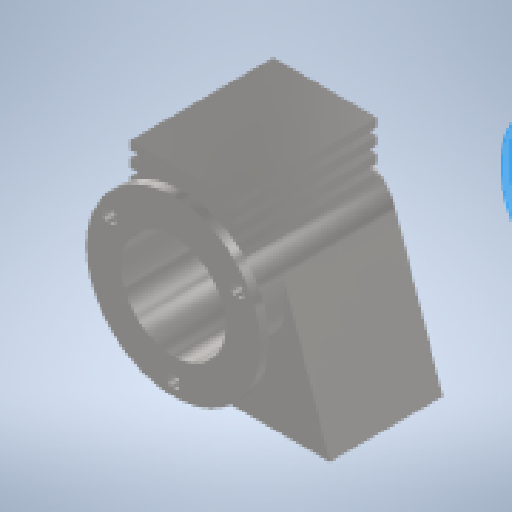
# Autodesk Inventor part: Base do Motor Industrial
Saved by Autodesk Inventor 2023.2 (Build 272271000, 271)
## iProperties
Created: 2022-07-18
Part Number: Base do Motor Industrial
Material: Steel, Carbon
Document SubType Name: Modeling
Designer: coqui
Density: 7.85 g/cm^3
Appearance: Semi-Polished
Mass: 4415.21 g
Surface Area: 866.573 cm^2
Volume: 562.447 cm^3
Author: coqui
Autodesk Inventor part; units mm, degrees
ref_plane "YZ Plane" through (0, 0, 0) normal (1, 0, 0) x (0, 1, 0)
ref_plane "XZ Plane" through (0, 0, 0) normal (0, 1, 0) x (-1, 0, 0)
ref_plane "XY Plane" through (0, 0, 0) normal (0, 0, 1) x (1, 0, 0)
sketch "Sketch1" plane through (0, 0, 0) normal (0, 0, 1) x (1, 0, 0)
  arc A0 (33.1265, 11.2976) -> (-33.1265, 11.2976) centre (0, 0) ccw
  line L0 (-60, -67.5) -> (60, -67.5)
  line L1 (-60, -67.5) -> (-33.1265, 11.2976)
  line L2 (60, -67.5) -> (33.1265, 11.2976)
  point P0 (0, -67.5)
  dimension "d0" = 70
  dimension "d1" = 120
  dimension "d2" = 60
  dimension "d3" = 67.5
  constraints: 6 end point, 2 point on circle, 2 tangent, 1 centre point, 1 coincident, 1 horizontal, 1 midpoint
  measures "d0" diameter of A0
  measures "d1" distance of L0.start L0.end
  measures "d2" horizontal distance of L0.end point (0, 0)
  measures "d3" distance of point (0, -67.5) point (0, 0)
extrude "Extrusion1" add sketch "Sketch1" along normal blind 65
sketch "Sketch2" plane through (0, 0, 65) normal (0, 0, 1) x (1, 0, 0)
  circle A0 centre (0, 0) radius 35
  dimension "d6" = 70
  constraints: 1 centre point, 1 coincident
  measures "d6" diameter of A0
extrude "Extrusion2" add sketch "Sketch2" along normal blind 25
sketch "Sketch3" plane through (0, 0, 90) normal (0, 0, 1) x (1, 0, 0)
  circle A0 centre (0, 0) radius 50
  dimension "d9" = 100
  constraints: 1 centre point, 1 coincident
  measures "d9" diameter of A0
extrude "Extrusion3" add sketch "Sketch3" along normal blind 5
sketch "Sketch4" plane through (0, 0, 95) normal (0, 0, 1) x (1, 0, 0)
  circle A0 centre (0, -42.5) radius 3.75
  circle A1 centre (36.8061, 21.25) radius 3.75
  circle A2 centre (-36.8061, 21.25) radius 3.75
  point P0 (0, 0)
  dimension "d12" = 7.5
  dimension "d13" = 42.5
  dimension "d16" = 360
  constraints: 3 centre point, 7 other
  measures "d12" diameter of A0
  measures "d13" distance of point (0, 0) A0.centre
extrude "Extrusion4" cut sketch "Sketch4" against normal blind 5
sketch "Sketch5" plane through (0, 0, 90) normal (0, 0, -1) x (-1, 0, 0)
  line L0 (0, 60) -> (-30, 60)
  line L1 (-30, 60) -> (-30, 55.5)
  line L2 (-30, 55.5) -> (-25, 55.5)
  line L3 (-25, 55.5) -> (-25, 51)
  line L4 (-25, 51) -> (-30, 51)
  line L5 (-30, 51) -> (-30, 46.5)
  line L6 (-30, 46.5) -> (-25, 46.5)
  line L7 (-25, 46.5) -> (-25, 42)
  line L8 (-25, 42) -> (-30, 42)
  line L9 (-30, 42) -> (-30, 37.5)
  line L10 (-30, 37.5) -> (-25, 37.5)
  line L11 (-25, 37.5) -> (-25, 33)
  line L12 (-25, 33) -> (-30, 33)
  line L13 (-30, 33) -> (-30, 28.5)
  line L14 (-30, 28.5) -> (-25, 28.5)
  line L15 (-25, 28.5) -> (-25, 24)
  line L16 (-25, 24) -> (-30, 24)
  line L17 (-30, 24) -> (-30, 19.5)
  line L18 (-30, 19.5) -> (-25, 19.5)
  arc A0 (33.1265, 11.2976) -> (-33.1265, 11.2976) centre (0, 0) ccw projected
  line L19 (-25, 19.5) -> (0, 19.5)
  line L20 (0, 60) -> (30, 60)
  line L21 (30, 60) -> (30, 55.5)
  line L22 (30, 55.5) -> (25, 55.5)
  line L23 (25, 55.5) -> (25, 51)
  line L24 (25, 51) -> (30, 51)
  line L25 (30, 51) -> (30, 46.5)
  line L26 (30, 46.5) -> (25, 46.5)
  line L27 (25, 46.5) -> (25, 42)
  line L28 (25, 42) -> (30, 42)
  line L29 (30, 42) -> (30, 37.5)
  line L30 (30, 37.5) -> (25, 37.5)
  line L31 (25, 37.5) -> (25, 33)
  line L32 (25, 33) -> (30, 33)
  line L33 (30, 33) -> (30, 28.5)
  line L34 (30, 28.5) -> (25, 28.5)
  line L35 (25, 28.5) -> (25, 24)
  line L36 (25, 24) -> (30, 24)
  line L37 (30, 24) -> (30, 19.5)
  line L38 (30, 19.5) -> (25, 19.5)
  line L39 (25, 19.5) -> (0, 19.5)
  point P0 (0, 35)
  point P1 (-25, 24.4949)
  point P2 (25, 24.4949)
  dimension "d20" = 4.5
  dimension "d21" = 4.5
  dimension "d22" = 4.5
  dimension "d23" = 4.5
  dimension "d24" = 4.5
  dimension "d25" = 4.5
  dimension "d26" = 4.5
  dimension "d27" = 4.5
  dimension "d29" = 5
  dimension "d30" = 5
  dimension "d31" = 4.5
  dimension "d32" = 30
  dimension "d34" = 60
  constraints: 80 end point, 26 point on line, 10 perpendicular, 3 horizontal, 1 point on circle
  measures "d20" distance of L0.end L1.end
  measures "d21" distance of L2.end L3.end
  measures "d22" distance of L4.end L5.end
  measures "d23" distance of L6.end L7.end
  measures "d24" distance of L8.end L9.end
  measures "d25" distance of L10.end L11.end
  measures "d26" distance of L12.end L13.end
  measures "d27" distance of L14.end L15.end
  measures "d29" distance of L2.end L1.end
  measures "d30" distance of L15.end L16.end
  measures "d31" distance of L16.end L17.end
  measures "d32" distance of L0.start L0.end
  measures "d34" vertical distance of point (0, 0) L0.end
extrude "Extrusion5" add sketch "Sketch5" along normal blind 82.5 contours L20 L21 L22 L23 L24 L25 L26 L27 L28 L29 L30 L31 L32 L33 L34 L35 A0 L15 L14 L13 L12 L11 L10 L9 L8 L7 L6 L5 L4 L3 L2 L1 L0
sketch "Sketch6" plane through (0, 0, 95) normal (0, 0, 1) x (1, 0, 0)
  circle A0 centre (0, 0) radius 30
  dimension "d38" = 60
  constraints: 1 centre point, 1 coincident
  measures "d38" diameter of A0
extrude "Extrusion6" cut sketch "Sketch6" against normal blind 90
sketch "Sketch7" plane through (0, 0, 5) normal (0, 0, 1) x (1, 0, 0)
  circle A0 centre (0, 0) radius 7.5
  dimension "d41" = 15
  constraints: 1 centre point, 1 coincident
  measures "d41" diameter of A0
extrude "Extrusion7" cut sketch "Sketch7" against normal blind 90
body "Solid1"
